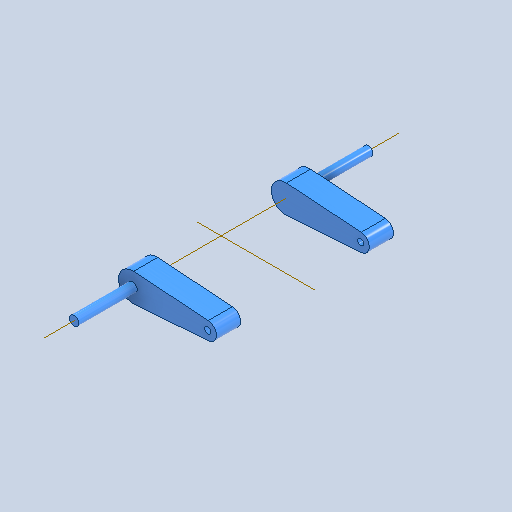
# Autodesk Inventor part: Type 1A R4主滑台曲柄:1
Saved by Autodesk Inventor 2025 (Build 290162000, 162)
## iProperties
Created: 2024-10-07
Part Number: Type 1A R4主滑台曲柄:1
Material: 密度7850的鋼
Document SubType Name: Modeling
Designer: user
Density: 7.84999 g/cm^3
Appearance: 青
Mass: 67383.1 g
Surface Area: 4297.68 cm^2
Volume: 8583.84 cm^3
Author: user
Autodesk Inventor part; units mm, degrees
ref_plane "YZ Plane" through (0, 0, 0) normal (1, 0, 0) x (0, 1, 0)
ref_plane "XZ Plane" through (0, 0, 0) normal (0, 1, 0) x (-1, 0, 0)
ref_plane "工作平面1" through (0, 0, 378) normal (0, 0, 1) x (1, 0, 0)
sketch "草圖1" plane through (0, 0, 378) normal (0, 0, 1) x (1, 0, 0)
  line L0 (0, 0) -> (320.6953, 0) construction
  circle A0 centre (0, 0) radius 60
  circle A1 centre (320.6953, 0) radius 37.5
  line L1 (4.2096, 59.8521) -> (323.3263, 37.4076)
  line L2 (4.2096, -59.8521) -> (323.3263, -37.4076)
  point P0 (-31.7926, 50.8845)
  dimension "d3" = 320.6953
  dimension "d4" = 120
  dimension "d6" = 75
  constraints: 6 end point, 5 point on circle, 4 tangent, 2 centre point, 2 coincident, 1 horizontal
  measures "d3" distance of L0.start L0.end
  measures "d4" diameter of A0
  measures "d6" diameter of A1
extrude "擠出1" add sketch "草圖1" against normal blind 103
sketch "草圖2" plane through (0, 0, 378) normal (0, 0, 1) x (1, 0, 0)
  arc A0 (4.2096, 59.8521) -> (4.2096, -59.8521) centre (0, 0) ccw projected
  arc A1 (323.3263, -37.4076) -> (323.3263, 37.4076) centre (320.6953, 0) ccw projected
  circle A2 centre (320.6953, 0) radius 13.25
  point P0 (70.7107, 70.7107)
  dimension "d13" = 26.5
  constraints: 1 centre point, 1 coincident
  measures "d13" diameter of A2
extrude "擠出2" cut sketch "草圖2" against normal through all
sketch "草圖8" plane through (0, 0, 378) normal (0, 0, 1) x (1, 0, 0)
  circle A0 centre (0, 0) radius 19.875
  dimension "d51" = 39.75
  constraints: 1 centre point, 1 coincident
  measures "d51" diameter of A0
extrude "擠出3" add sketch "草圖8" along normal blind 250
sketch "草圖3" plane through (323.3263, 37.4076, 378) normal (0.0701601, 0.9975357, 0) x (0.9975357, -0.0701601, 0)
  line L0 (0, 0) -> (0, 103) projected
  point P0 (-319.905, 378)
  point P1 (0, 51.5)
  constraints: 1 midpoint
hole "孔1" [suppressed]
sketch "草圖5" plane through (11.1138, -59.3666, 275) normal (-0.0701601, 0.9975357, 0) x (0, 0, 1)
  line L0 (103, 312.9838) -> (0, 312.9838) projected
  point P0 (-275, -6.9212)
  point P1 (51.5, 312.9838)
  constraints: 1 midpoint
hole "孔3" [suppressed]
mirror "鏡射1" about plane through (0, 0, 0) normal (0, 0, 1) of "擠出1", "擠出2", "擠出3"
equation "\"d3\" = R4"
equation "\"R4\" = T1A_R4"
equation "\"th4a\" = T1A_th4a"
equation "\"Width\" = T1A_R4_Width"
equation "\"d0\" = 0.5 * Width"
equation "\"T1A_R4\" = 320.6953"
equation "\"T1A_th4a\" = 45deg"
equation "\"T1A_R4_Width\" = 756"
equation "\"T1A_R1\" = 585.5331"
equation "\"T1A_R3\" = 252.3048"
equation "\"T1A_R5\" = 419.3047"
equation "\"T1A_R7\" = -221.7475"
equation "\"T1A_R8\" = 369.2781"
equation "\"T1A_R1_Width\" = 756"
equation "\"T1A_R2_Width\" = 756"
equation "\"T1A_R3_Width\" = 344"
equation "\"T1A_Joint_Width\" = 756"
